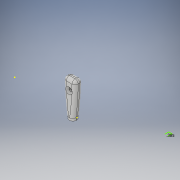
# Autodesk Inventor part: dis3
Saved by Autodesk Inventor 2018 (Build 220112000, 112)
## iProperties
Created: 2019-04-29
Part Number: dis3
Material: Generic
Document SubType Name: Modeling
Designer: 10043883
Density: 1 g/cm^3
Appearance: Default
Author: 10043883
Autodesk Inventor part; units mm, degrees
ref_plane "YZ Plane" through (0, 0, 0) normal (1, 0, 0) x (0, 1, 0)
ref_plane "XZ Plane" through (0, 0, 0) normal (0, 1, 0) x (-1, 0, 0)
ref_plane "XY Plane" through (0, 0, 0) normal (0, 0, 1) x (1, 0, 0)
sketch "Sketch1" plane through (0, 0, 0) normal (0, 0, 1) x (1, 0, 0)
  line L0 (138.6197, 0) -> (167.8932, 0)
  line L1 (144.3665, -82.6516) -> (162.1465, -82.6516)
  arc A0 (162.1465, -82.6516) -> (167.8932, 0) centre (-429.3411, 0) ccw
  arc A1 (138.6197, 0) -> (144.3665, -82.6516) centre (735.854, 0) ccw
  point P0 (0, 0)
  point P1 (161.6207, -82.6516)
  point P2 (153.734, -82.6516)
  dimension "d0" = 29.2735
  dimension "d2" = 17.78
  constraints: 4 end point, 4 point on circle, 4 point on line, 3 horizontal, 2 centre point, 1 equal radius
  measures "d0" distance of L0.start L0.end
  measures "d2" distance of L1.start L1.end
extrude "Extrusion1" add sketch "Sketch1" along normal blind 18.7706
fillet "Fillet1" radius 7.62 8 edges at (140.0581, -41.4256, 18.7706) (166.4548, -41.4256, 18.7706) (153.2565, 0, 18.7706) (153.2565, 0, 0) (138.6197, 0, 9.3853) (167.8932, 0, 9.3853) (140.0581, -41.4256, 0) (166.4548, -41.4256, 0)
sketch "Sketch2" plane through (152.0615, -82.6516, 18.7706) normal (0, -1, 0) x (1, 0, 0)
  line L0 (161.6207, -82.6516) -> (161.6207, -92.4306)
  line L1 (153.734, -92.4306) -> (153.734, -82.6516)
  line L2 (161.6207, -92.4306) -> (153.734, -92.4306)
  line L3 (10.085, -11.1506) -> (10.085, -7.62) projected
  line L4 (10.085, -9.3853) -> (-7.695, -9.3853)
  line L5 (-7.695, -11.1506) -> (-7.695, -7.62) projected
  point P0 (-152.0615, -18.7706)
  dimension "d10" = 9.779
  constraints: 8 end point, 2 midpoint, 1 vertical
  measures "d10" distance of L0.start L2.start
ref_plane "Work Plane1" through (162.1465, -82.6516, 9.3853) normal (0, 0, 1) x (-1, 0, 0)
sketch "Sketch3" plane through (162.1465, -82.6516, 9.3853) normal (0, 0, 1) x (-1, 0, 0)
  arc A0 (0, 0) -> (-5.6969, -74.9331) centre (591.4875, -82.6516) ccw projected
  line L0 (0, 5.7277) -> (0, 0)
  arc A1 (0, 0) -> (-5.6969, -74.9331) centre (591.4875, -82.6516) ccw projected
  line L1 (-5.6969, -74.9331) -> (8.89, 0)
  line L2 (8.89, 0) -> (8.89, 5.7277)
  line L3 (0, 5.7277) -> (8.89, 5.7277)
  line L4 (8.89, 0) -> (0, 0)
  point P0 (162.1465, -82.6516)
  dimension "d14" = 76.3397
  constraints: 10 end point, 1 horizontal, 1 parallel
  measures "d14" distance of L1.start L1.end
revolve "Revolution2" add sketch "Sketch3" angle 360 about axis through (153.2565, -82.6516, 9.3853) along (0, -1, 0) contours L0 L3 L2 L4
sketch "Sketch4" plane through (153.2565, -88.3793, 9.3853) normal (0, -1, 0) x (1, 0, 0)
  circle A0 centre (0, 0) radius 5.207
  circle A1 centre (0, 0) radius 8.89 projected
  line L0 (-5.1798, 0.5316) -> (-8.697, 0.5316)
  line L1 (-8.697, 0.5316) -> (-8.697, -0.7384)
  line L2 (-8.697, -0.7384) -> (-5.1798, -0.7384)
  line L3 (-5.1798, -0.7384) -> (-5.1798, 0.5316)
  line L4 (5.1798, 0.5316) -> (8.697, 0.5316)
  line L5 (8.697, 0.5316) -> (8.697, -0.7384)
  line L6 (8.697, -0.7384) -> (5.1798, -0.7384)
  line L7 (5.1798, -0.7384) -> (5.1798, 0.5316)
  point P0 (-153.2565, -9.3853)
  dimension "d17" = 3.683
  dimension "d18" = 1.27
  constraints: 16 end point, 2 parallel, 1 horizontal, 1 perpendicular, 4 other
  measures "d18" distance of L1.end L0.end
extrude "Extrusion2" cut sketch "Sketch4" against normal blind 16.2306 contours A0 L7 | A0 L4 L5 L6 L7 | L7 A0 L3 | L3 A0 | A0 L3 L2 L1 L0
sketch "Sketch5" plane through (0, 0, 18.7706) normal (0, 0, 1) x (1, 0, 0)
  line L0 (160.224, 0) -> (146.289, 0) projected
  line L1 (152.6894, 0) -> (178.0894, 0) construction
  circle A0 centre (152.6894, -25.4) radius 8.3376
  point P0 (0, 0)
  dimension "d23" = 16.6751
  constraints: 2 end point, 1 centre point, 1 horizontal, 1 point on line
  measures "d23" diameter of A0
hole "Hole1" at (152.6894, -25.4, 18.7706) direction (0, 0, -1) diameter 8.382 end through all countersink diameter 16.383 countersink angle 82
sketch "Sketch6" plane through (0, 0, 0) normal (0, 0, -1) x (-1, 0, 0)
  line L0 (-160.224, 0) -> (-146.289, 0) projected
  line L1 (-153.2565, 0) -> (-152.7232, -25.4729)
  point P0 (0, 0)
  constraints: 2 end point, 1 midpoint
hole "Hole2" at (152.7232, -25.4729, 0) direction (0, 0, 1) diameter 8.382 end through all countersink diameter 17.9705 countersink angle 82
body "Solid1"
